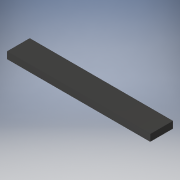
# Autodesk Inventor part: socket_pcb
Saved by Autodesk Inventor 2018 (Build 220112000, 112)
## iProperties
Created: 2018-12-04
Part Number: socket_pcb
Material: Generic
Document SubType Name: Modeling
Designer: jaspe
Density: 1 g/cm^3
Appearance: Default
Author: jaspe
Autodesk Inventor part; units mm, degrees
ref_plane "YZ Plane" through (0, 0, 0) normal (1, 0, 0) x (0, 1, 0)
ref_plane "XZ Plane" through (0, 0, 0) normal (0, 1, 0) x (-1, 0, 0)
ref_plane "XY Plane" through (0, 0, 0) normal (0, 0, 1) x (1, 0, 0)
sketch "Sketch1" plane through (0, 0, 0) normal (0, 1, 0) x (-1, 0, 0)
  line L0 (-27, 1.27) -> (27, 1.27)
  line L1 (27, 1.27) -> (27, -1.27)
  line L2 (27, -1.27) -> (-27, -1.27)
  line L3 (-27, -1.27) -> (-27, 1.27)
  line L4 (-27, 1.27) -> (27, -1.27) construction
  line L5 (27, 1.27) -> (-27, -1.27) construction
  point P0 (0, 0)
  dimension "d0" = 54
  dimension "d1" = 2.54
  constraints: 12 end point, 2 midpoint, 2 parallel, 1 horizontal, 1 perpendicular
  measures "d0" distance of L1.end L2.end
  measures "d1" distance of L0.end L1.end
extrude "Extrusion1" add sketch "Sketch1" along normal blind 8.5
body "Solid1"
